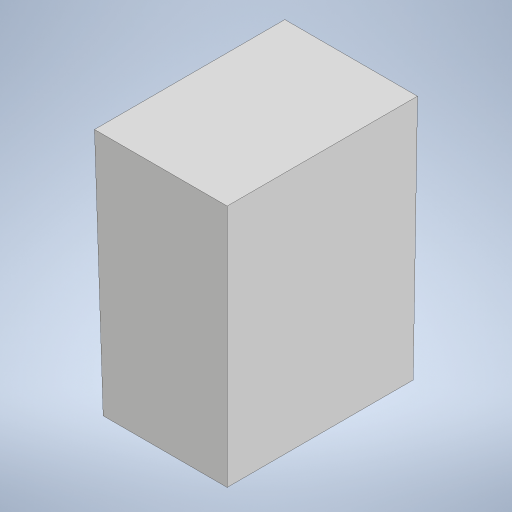
# Autodesk Inventor part: Cylinder Cast Image
Saved by Autodesk Inventor 2023 (Build 270158000, 158)
## iProperties
Created: 2022-12-28
Part Number: Cylinder Cast Image
Material: Generic
Document SubType Name: Modeling
Designer: tgr41
Density: 1 g/cm^3
Appearance: Default
Author: tgr41
Autodesk Inventor part; units mm, degrees
ref_plane "YZ Plane" through (0, 0, 0) normal (1, 0, 0) x (0, 1, 0)
ref_plane "XZ Plane" through (0, 0, 0) normal (0, 1, 0) x (-1, 0, 0)
ref_plane "XY Plane" through (0, 0, 0) normal (0, 0, 1) x (1, 0, 0)
sketch "Sketch1" plane through (0, 0, 0) normal (0, 1, 0) x (-1, 0, 0)
  circle A0 centre (3.4811, 6.9947) radius 6.35
  line L0 (-9.2189, 19.6947) -> (16.1811, 19.6947)
  line L1 (16.1811, 19.6947) -> (16.1811, -18.4053)
  line L2 (16.1811, -18.4053) -> (-9.2189, -18.4053)
  line L3 (-9.2189, -18.4053) -> (-9.2189, 19.6947)
  point P0 (0, 0)
  dimension "d0" = 12.7
  dimension "d1" = 25.4
  dimension "d2" = 38.1
  dimension "d3" = 12.7
  dimension "d4" = 12.7
  constraints: 8 end point, 2 parallel, 1 centre point, 1 horizontal, 1 perpendicular
  measures "d0" diameter of A0
  measures "d1" distance of L1.end L2.end
  measures "d2" distance of L0.end L1.end
  measures "d3" distance from line of L3 A0.centre
  measures "d4" distance from line of A0.centre L0
extrude "Extrusion1" add sketch "Sketch1" along normal blind 50.8 contours A0 | L0 L1 L2 L3
extrude "Extrusion2" cut sketch "Sketch1" along normal blind 44.45 contours A0
draft "FaceDraft1" angle 1 pull direction (0, -1, 0) faces at (9.2189, 16.9333, 6.9947) (-16.1811, 16.9333, -5.7053) (-7.7145, 33.8667, 19.6947) (-9.7489, 29.6333, 5.9761) fixed edges at (9.2189, 0, 0.6447) (-16.1811, 0, 0.6447) (-3.4811, 0, 19.6947) (2.8689, 0, 6.9947)
body "Solid1"
